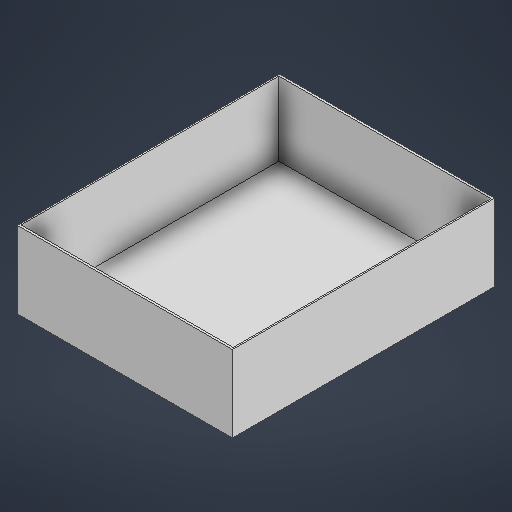
# Autodesk Inventor part: Pelican box
Saved by Autodesk Inventor 2026.1 (Build 301233020, 233B)
## iProperties
Created: 2025-09-30
Part Number: Pelican box
Material: Generic
Document SubType Name: Modeling
Designer: maria
Density: 1 g/cm^3
Appearance: Default
Author: maria
Autodesk Inventor part; units mm, degrees
ref_plane "YZ Plane" through (0, 0, 0) normal (1, 0, 0) x (0, 1, 0)
ref_plane "XZ Plane" through (0, 0, 0) normal (0, 1, 0) x (-1, 0, 0)
ref_plane "XY Plane" through (0, 0, 0) normal (0, 0, 1) x (1, 0, 0)
sketch "Sketch1" plane through (0, 0, 0) normal (0, 1, 0) x (-1, 0, 0)
  line L0 (-231.775, 282.575) -> (231.775, 282.575)
  line L1 (231.775, 282.575) -> (231.775, -282.575)
  line L2 (231.775, -282.575) -> (-231.775, -282.575)
  line L3 (-231.775, -282.575) -> (-231.775, 282.575)
  line L4 (-231.775, 282.575) -> (231.775, -282.575) construction
  line L5 (231.775, 282.575) -> (-231.775, -282.575) construction
  point P0 (0, 0)
  dimension "d0" = 565.15
  dimension "d1" = 463.55
  constraints: 12 end point, 2 midpoint, 2 parallel, 1 horizontal, 1 perpendicular
  measures "d0" distance of L0.end L1.end
  measures "d1" distance of L1.end L2.end
extrude "Extrusion1" add sketch "Sketch1" along normal blind 158.75 and the other way blind 6.35
sketch "Sketch2" plane through (0, 158.75, 0) normal (0, 1, 0) x (1, 0, 0)
  line L0 (228.6, -277.8125) -> (-228.6, -277.8125)
  line L1 (-228.6, -277.8125) -> (-228.6, 277.8125)
  line L2 (-228.6, 277.8125) -> (228.6, 277.8125)
  line L3 (228.6, 277.8125) -> (228.6, -277.8125)
  line L4 (228.6, -277.8125) -> (-228.6, 277.8125) construction
  line L5 (-228.6, -277.8125) -> (228.6, 277.8125) construction
  point P0 (0, 0)
  dimension "d4" = 555.625
  dimension "d5" = 457.2
  constraints: 12 end point, 2 midpoint, 2 parallel, 1 horizontal, 1 perpendicular
  measures "d4" distance of L0.end L1.end
  measures "d5" distance of L1.end L2.end
extrude "Extrusion2" cut sketch "Sketch2" against normal blind 158.75
body "Solid1"
